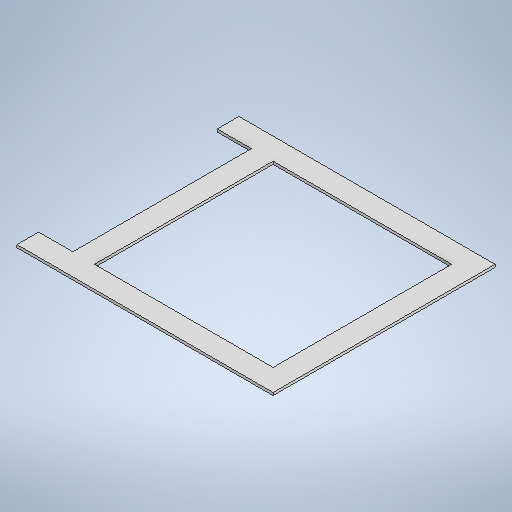
# Autodesk Inventor part: Metal2
Saved by Autodesk Inventor 2025 (Build 290162000, 162)
## iProperties
Created: 2024-11-07
Part Number: Metal2
Material: Generic
Document SubType Name: Sheet Metal
Designer: g.marin
Density: 1 g/cm^3
Sheet Metal Rule: Default
Appearance: Default
Author: g.marin
Autodesk Inventor part; units mm, degrees
ref_plane "YZ Plane" through (0, 0, 0) normal (1, 0, 0) x (0, 1, 0)
ref_plane "XZ Plane" through (0, 0, 0) normal (0, 1, 0) x (-1, 0, 0)
ref_plane "XY Plane" through (0, 0, 0) normal (0, 0, 1) x (1, 0, 0)
sketch "Sketch1" plane through (0, 0, 0) normal (0, 1, 0) x (-1, 0, 0)
  line L0 (-130, 130) -> (130, 130)
  line L1 (130, 130) -> (130, -130)
  line L2 (130, -130) -> (-130, -130)
  line L3 (-130, -130) -> (-130, 130)
  line L4 (-130, 130) -> (130, -130) construction
  line L5 (130, 130) -> (-130, -130) construction
  line L6 (-104.6, 104.6) -> (104.6, 104.6)
  line L7 (104.6, 104.6) -> (104.6, -104.6)
  line L8 (104.6, -104.6) -> (-104.6, -104.6)
  line L9 (-104.6, -104.6) -> (-104.6, 104.6)
  line L10 (-104.6, 104.6) -> (104.6, -104.6) construction
  line L11 (104.6, 104.6) -> (-104.6, -104.6) construction
  line L12 (130, 130) -> (170, 130)
  line L13 (170, 130) -> (170, 104.6)
  line L14 (170, 104.6) -> (130, 104.6)
  line L15 (130, 104.6) -> (130, 130)
  line L16 (130, -130) -> (170, -130)
  line L17 (170, -130) -> (170, -104.6)
  line L18 (170, -104.6) -> (130, -104.6)
  line L19 (130, -104.6) -> (130, -130)
  point P0 (0, 0)
  dimension "d0" = 260
  dimension "d1" = 260
  dimension "d2" = 25.4
  dimension "d3" = 40
  constraints: 40 end point, 8 parallel, 4 horizontal, 4 midpoint, 4 perpendicular, 2 collinear, 2 point on line
  measures "d0" distance of L0.end L1.end
  measures "d1" distance of L0.start L0.end
  measures "d2" distance between parallel lines of L6 L0
  measures "d3" distance between parallel lines of L15 L13
extrude "Extrusion1" add sketch "Sketch1" along normal blind 3.175
equation "\"BendRadius\" = Thickness"
equation "\"BendReliefWidth\" = Thickness"
equation "\"BendReliefDepth\" = 0.5 * Thickness"
equation "\"CornerReliefSize\" = 4 * Thickness"
equation "\"MinimumRemnant\" = 2 * Thickness"
equation "\"TransitionRadius\" = BendRadius"
equation "\"JacobiRadiusSize\" = BendRadius"
equation "\"GapSize\" = Thickness"
equation "\"Thickness\" = 3.048"
body "Solid1"
